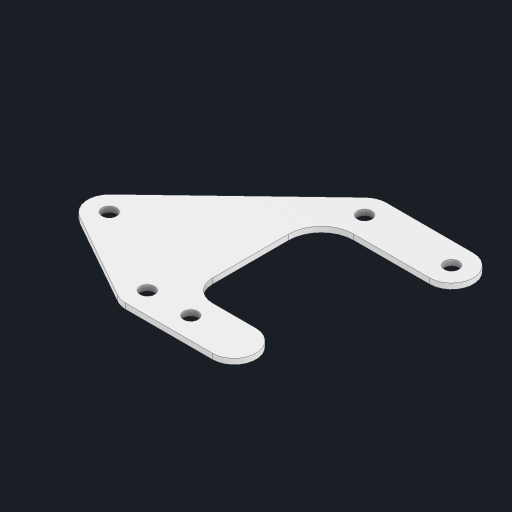
# Autodesk Inventor part: gusset
Saved by Autodesk Inventor 2024 (Build 280153000, 153)
## iProperties
Created: 2024-03-11
Part Number: gusset
Material: Acetal Resin, White
Document SubType Name: Modeling
Designer: Averey Ku
Density: 1.425 g/cm^3
Appearance: Smooth - White
Author: Averey Ku
Autodesk Inventor part; units mm, degrees
ref_plane "YZ Plane" through (0, 0, 0) normal (1, 0, 0) x (0, 1, 0)
ref_plane "XZ Plane" through (0, 0, 0) normal (0, 1, 0) x (-1, 0, 0)
ref_plane "XY Plane" through (0, 0, 0) normal (0, 0, 1) x (1, 0, 0)
sketch "main" plane through (0, 0, 0) normal (0, 0, 1) x (1, 0, 0)
  arc A0 (-6.1043, -28.9805) -> (-1.6752, -27.2152) centre (-6.0688, -22.6306) ccw
  arc A1 (-31.4687, -16.2806) -> (-31.4687, -28.9806) centre (-31.4688, -22.6306) ccw
  circle A2 centre (-6.0688, -22.6306) radius 2.0955
  circle A3 centre (-31.4688, -22.6306) radius 2.0955
  arc A4 (-9.2438, -16.2806) -> (0.2812, -6.7556) centre (-9.2438, -6.7556) ccw
  line L0 (-9.2438, -16.2806) -> (-31.4688, -16.2806)
  line L1 (-6.0331, -28.9805) -> (-31.4687, -28.9806)
  circle A5 centre (-6.0688, 28.169) radius 2.0955
  circle A6 centre (6.6312, 28.1694) radius 2.0955
  arc A7 (9.7441, 33.7036) -> (6.6312, 34.519) centre (6.6312, 28.1694) ccw
  line L2 (0.2812, 15.4694) -> (0.2812, -6.7556)
  line L3 (36.4248, 9.2973) -> (-1.6752, -27.2152)
  line L4 (-18.7688, 21.8194) -> (-6.0688, 21.8194)
  arc A8 (0.2812, 15.4694) -> (-6.0688, 21.8194) centre (-6.0688, 15.4694) ccw
  arc A9 (-18.6975, 34.519) -> (-18.7688, 21.8194) centre (-18.7688, 28.1694) ccw
  line L5 (-18.6975, 34.519) -> (6.6312, 34.519)
  circle A10 centre (32.0312, 13.8819) radius 2.0955
  arc A11 (36.4248, 9.2973) -> (35.1443, 19.4165) centre (32.0312, 13.8819) ccw
  line L6 (9.7441, 33.7036) -> (35.1443, 19.4165)
  point P0 (-4.0049, 2.2465)
  dimension "d0" = 4.191
  dimension "d1" = 4.191
  dimension "d2" = 12.7
  dimension "d3" = 9.525
  dimension "d4" = 6.35
  measures "d0" diameter of A5
  measures "d1" diameter of A10
  measures "d2" diameter of A0
  measures "d3" radius of A4
  measures "d4" radius of A8
sketch "Sketch1" plane through (0, 0, 0) normal (0, 1, 0) x (-1, 0, 0)
  arc A0 (-0.0356, -57.1495) -> (4.3936, -55.3842) centre (0, -50.7996) ccw
  arc A1 (-25.4, -44.4496) -> (-25.4, -57.1496) centre (-25.4, -50.7996) ccw
  circle A2 centre (0, -50.7996) radius 2.0955
  circle A3 centre (-25.4, -50.7996) radius 2.0955
  arc A4 (-3.175, -44.4496) -> (6.35, -34.9246) centre (-3.175, -34.9246) ccw
  line L0 (-3.175, -44.4496) -> (-25.4, -44.4496)
  line L1 (0.0356, -57.1495) -> (-25.4, -57.1496)
  circle A5 centre (0, 0) radius 2.0955
  circle A6 centre (12.7, 0.0004) radius 2.0955
  arc A7 (15.8129, 5.5346) -> (12.7, 6.35) centre (12.7, 0.0004) ccw
  line L2 (6.35, -12.6996) -> (6.35, -34.9246)
  line L3 (42.4936, -18.8717) -> (4.3936, -55.3842)
  line L4 (-12.7, -6.3496) -> (0, -6.3496)
  arc A8 (6.35, -12.6996) -> (0, -6.3496) centre (0, -12.6996) ccw
  arc A9 (-12.6287, 6.35) -> (-12.7, -6.3496) centre (-12.7, 0.0004) ccw
  line L5 (-12.6287, 6.35) -> (12.7, 6.35)
  circle A10 centre (38.1, -14.2871) radius 2.0955
  arc A11 (42.4936, -18.8717) -> (41.2131, -8.7526) centre (38.1, -14.2871) ccw
  line L6 (15.8129, 5.5346) -> (41.2131, -8.7526)
  constraints: 1 other
extrude "Extrusion1" add sketch "Sketch1" along normal blind 1.5875
body "Solid1"
